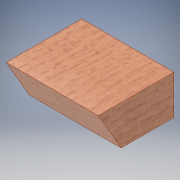
# Autodesk Inventor part: BA02
Saved by Autodesk Inventor 2017 (Build 210142000, 142)
## iProperties
Created: 2018-10-17
Part Number: BA02
Material: Wood (Oak)
Document SubType Name: Modeling
Designer: Administrator
Density: 0.76 g/cm^3
Appearance: White Oak - Natural Medium Gloss
Author: Administrator
Autodesk Inventor part; units mm, degrees
ref_plane "YZ Plane" through (0, 0, 0) normal (1, 0, 0) x (0, 1, 0)
ref_plane "XZ Plane" through (0, 0, 0) normal (0, 1, 0) x (-1, 0, 0)
ref_plane "XY Plane" through (0, 0, 0) normal (0, 0, 1) x (1, 0, 0)
sketch "Sketch1" plane through (0, 0, 0) normal (0, 0, 1) x (1, 0, 0)
  line L0 (0, 0) -> (88.9, 0)
  line L1 (88.9, 0) -> (88.9, 38.1)
  line L2 (88.9, 38.1) -> (0, 38.1)
  line L3 (0, 38.1) -> (0, 0)
  dimension "d0" = 88.9
  dimension "d1" = 38.1
  constraints: 8 end point, 2 parallel, 1 horizontal, 1 perpendicular
  measures "d0" distance of L2.end L1.end
  measures "d1" distance between parallel lines of L0 L2
extrude "Extrusion1" add sketch "Sketch1" along normal blind 50.8
sketch "Sketch2" plane through (88.9, 0, 0) normal (1, 0, 0) x (0, 0, -1)
  line L0 (-50.8, 0) -> (-72.797, 38.1)
  line L1 (-50.8, 0) -> (-50.8, 38.1) projected
  line L2 (-72.797, 38.1) -> (-50.8, 38.1)
  point P0 (0, 0)
  dimension "d4" = 30
  constraints: 4 end point, 1 perpendicular
  measures "d4" angle of L1 L0
extrude "Extrusion2" add sketch "Sketch2" against normal blind 88.9
body "Solid1"
